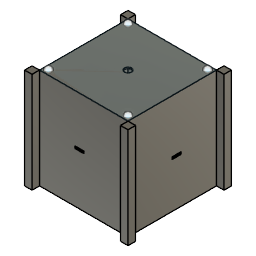
Hackathon Submission (Autodesk Fusion 360 design; units mm, degrees)
part number: 2026-03-29-19-09-48-508
Autodesk Fusion 360 part; units mm, degrees
sketch "Sketch1" plane through (0, 0, 0) normal (0, 0, 1) x (1, 0, 0)
  line L0 (0, 0) -> (100, 0)
  line L1 (100, 0) -> (100, 100)
  line L2 (100, 100) -> (0, 100)
  line L3 (0, 100) -> (0, 0)
  dimension "d1" = 100
  dimension "d2" = 100
  constraint horizontal L0
  constraint vertical L1
  constraint horizontal L2
  constraint vertical L3
  constraint coincident L0.start L3.end
  measures "d1" distance of L0.start L0.end
  measures "d2" distance of L0.start L2.end
extrude "Extrude1" add sketch "Sketch1" against normal blind 113.5
shell "Shell1" thickness 1.5 removed faces 1 at (33.3333, 66.6667, -113.5)
sketch "Sketch2" plane through (0, 0, 0) normal (0, 0, 1) x (1, 0, 0)
  line L0 (0, 0) -> (-8.5, 0)
  line L1 (-8.5, 0) -> (-8.5, -8.5)
  line L2 (-8.5, -8.5) -> (0, -8.5)
  line L3 (0, -8.5) -> (0, 0)
  line L4 (0, 100) -> (-8.5, 100)
  line L5 (-8.5, 100) -> (-8.5, 108.5)
  line L6 (-8.5, 108.5) -> (0, 108.5)
  line L7 (0, 108.5) -> (0, 100)
  line L8 (100, 100) -> (108.5, 100)
  line L9 (108.5, 100) -> (108.5, 108.5)
  line L10 (108.5, 108.5) -> (100, 108.5)
  line L11 (100, 108.5) -> (100, 100)
  line L12 (100, 0) -> (108.5, 0)
  line L13 (108.5, 0) -> (108.5, -8.5)
  line L14 (108.5, -8.5) -> (100, -8.5)
  line L15 (100, -8.5) -> (100, 0)
  dimension "d6" = 8.5
  dimension "d7" = 8.5
  dimension "d8" = 8.5
  dimension "d9" = 8.5
  dimension "d10" = 8.5
  dimension "d11" = 8.5
  dimension "d12" = 8.5
  dimension "d13" = 8.5
  constraint horizontal L0
  constraint vertical L1
  constraint horizontal L2
  constraint vertical L3
  constraint coincident L0.start L3.end
  constraint horizontal L4
  constraint vertical L5
  constraint horizontal L6
  constraint vertical L7
  constraint horizontal L8
  constraint vertical L9
  constraint horizontal L10
  constraint vertical L11
  constraint horizontal L12
  constraint vertical L13
  constraint horizontal L14
  constraint vertical L15
  measures "d6" distance of L0.start L0.end
  measures "d7" distance of L0.start L2.end
  measures "d8" distance of L4.start L4.end
  measures "d9" distance of L4.start L6.end
  measures "d10" distance of L8.start L8.end
  measures "d11" distance of L8.start L10.end
  measures "d12" distance of L12.start L12.end
  measures "d13" distance of L12.start L14.end
extrude "Extrude2" add sketch "Sketch2" against normal blind 113.5
sketch "Sketch3" plane through (100, 0, 0) normal (1, 0, 0) x (0, 1, 0)
  line L0 (100, 0) -> (0, 0)
  line L1 (0, 0) -> (0, -113.5)
  line L2 (0, -113.5) -> (100, -113.5)
  line L3 (100, -113.5) -> (100, 0)
  line L4 (50, -60) -> (60, -60)
  line L5 (60, -60) -> (60, -62.5)
  line L6 (60, -62.5) -> (50, -62.5)
  line L7 (50, -62.5) -> (50, -60)
  dimension "d16" = 10
  dimension "d17" = 2.5
  constraint horizontal L4
  constraint vertical L5
  constraint horizontal L6
  constraint vertical L7
  measures "d16" distance of L4.start L4.end
  measures "d17" distance of L4.start L6.end
extrude "Extrude3" cut sketch "Sketch3" against normal blind 10 contours L4 L5 L6 L7
sketch "Sketch4" plane through (0, 0, 0) normal (-1, 0, 0) x (0, -1, 0)
  line L0 (0, 0) -> (-100, 0)
  line L1 (-100, 0) -> (-100, -113.5)
  line L2 (-100, -113.5) -> (0, -113.5)
  line L3 (0, -113.5) -> (0, 0)
  line L4 (-50, -60) -> (-40, -60)
  line L5 (-40, -60) -> (-40, -62.5)
  line L6 (-40, -62.5) -> (-50, -62.5)
  line L7 (-50, -62.5) -> (-50, -60)
  dimension "d20" = 10
  dimension "d21" = 2.5
  constraint horizontal L4
  constraint vertical L5
  constraint horizontal L6
  constraint vertical L7
  measures "d20" distance of L4.start L4.end
  measures "d21" distance of L4.start L6.end
extrude "Extrude4" cut sketch "Sketch4" against normal blind 10 contours L4 L5 L6 L7
sketch "Sketch5" plane through (0, 100, 0) normal (0, 1, 0) x (-1, 0, 0)
  line L0 (0, 0) -> (-100, 0)
  line L1 (-100, 0) -> (-100, -113.5)
  line L2 (-100, -113.5) -> (0, -113.5)
  line L3 (0, -113.5) -> (0, 0)
  line L4 (-50, -60) -> (-60, -60)
  line L5 (-60, -60) -> (-60, -57.5)
  line L6 (-60, -57.5) -> (-50, -57.5)
  line L7 (-50, -57.5) -> (-50, -60)
  dimension "d24" = 10
  dimension "d25" = 2.5
  constraint horizontal L4
  constraint vertical L5
  constraint horizontal L6
  constraint vertical L7
  measures "d24" distance of L4.start L4.end
  measures "d25" distance of L4.start L6.end
extrude "Extrude5" cut sketch "Sketch5" against normal blind 10 contours L4 L5 L6 L7
sketch "Sketch6" plane through (0, 0, 0) normal (0, -1, 0) x (1, 0, 0)
  line L0 (100, 0) -> (0, 0)
  line L1 (0, 0) -> (0, -113.5)
  line L2 (0, -113.5) -> (100, -113.5)
  line L3 (100, -113.5) -> (100, 0)
  line L4 (50.0197, -56.75) -> (40.0197, -56.75)
  line L5 (40.0197, -56.75) -> (40.0197, -54.25)
  line L6 (40.0197, -54.25) -> (50.0197, -54.25)
  line L7 (50.0197, -54.25) -> (50.0197, -56.75)
  dimension "d28" = 10
  dimension "d29" = 2.5
  constraint horizontal L4
  constraint vertical L5
  constraint horizontal L6
  constraint vertical L7
  measures "d28" distance of L4.start L4.end
  measures "d29" distance of L4.start L6.end
extrude "Extrude6" cut sketch "Sketch6" against normal blind 10 contours L4 L5 L6 L7
sketch "Sketch7" plane through (0, 0, 0) normal (0, 0, 1) x (-1, 0, 0)
  line L0 (0, -100) -> (0, 0)
  line L1 (0, 0) -> (-100, 0)
  line L2 (-100, 0) -> (-100, -100)
  line L3 (-100, -100) -> (0, -100)
  circle A0 centre (-50, -50) radius 4
  dimension "d32" = 8
  measures "d32" diameter of A0
extrude "Extrude7" cut sketch "Sketch7" against normal blind 113.5 contours A0
sketch "Sketch8" plane through (0, 0, 0) normal (0, 0, 1) x (-1, 0, 0)
  circle A0 centre (-50, -50) radius 4
  line L0 (0, -100) -> (0, 0)
  line L1 (0, 0) -> (-100, 0)
  line L2 (-100, 0) -> (-100, -100)
  line L3 (-100, -100) -> (0, -100)
  circle A1 centre (-5, -5) radius 1.25
  dimension "d35" = 2.5
  measures "d35" diameter of A1
sketch "Sketch9" plane through (0, 0, 0) normal (0, 0, 1) x (-1, 0, 0)
  circle A0 centre (-5, -95) radius 1.25
  circle A1 centre (-95, -95) radius 1.25
  circle A2 centre (-95, -5) radius 1.25
  dimension "d36" = 2.5
  dimension "d37" = 2.5
  dimension "d38" = 2.5
  measures "d36" diameter of A0
  measures "d37" diameter of A1
  measures "d38" diameter of A2
